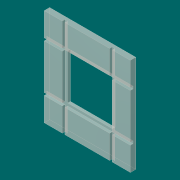
# Autodesk Inventor part: back
Saved by Autodesk Inventor 2016 (Build 200138000, 138)
## iProperties
Created: 2015-10-13
Part Number: back
Material: PC/ABS Plastic
Document SubType Name: Modeling
Designer: Sawaiz
Density: 0.357273 g/cm^3
Appearance: Clear
Author: Sawaiz
Autodesk Inventor part; units mm, degrees
ref_plane "YZ Plane" through (0, 0, 0) normal (1, 0, 0) x (0, 1, 0)
ref_plane "XZ Plane" through (0, 0, 0) normal (0, 1, 0) x (-1, 0, 0)
ref_plane "XY Plane" through (0, 0, 0) normal (0, 0, 1) x (1, 0, 0)
sketch "Sketch1" plane through (0, 0, 0) normal (1, 0, 0) x (0, 1, 0)
  line L0 (-50, -56.35) -> (50, -56.35)
  line L1 (50, -56.35) -> (50, 56.35)
  line L2 (50, 56.35) -> (-50, 56.35)
  line L3 (-50, 56.35) -> (-50, -56.35)
  line L4 (-50, -56.35) -> (50, 56.35) construction
  line L5 (50, -56.35) -> (-50, 56.35) construction
  point P0 (0, 0)
  dimension "d0" = 100
  dimension "d1" = 112.7
  constraints: 12 end point, 2 midpoint, 2 parallel, 1 horizontal, 1 perpendicular
  measures "d0" distance of L2.end L1.end
  measures "d1" distance of L1.end L0.end
extrude "Extrusion1" add sketch "Sketch1" along normal blind 6.35
sketch "Sketch2" plane through (6.35, 0, 0) normal (1, 0, 0) x (0, 0, -1)
  line L0 (-26, 26) -> (26, 26)
  line L1 (26, 26) -> (26, -26)
  line L2 (26, -26) -> (-26, -26)
  line L3 (-26, -26) -> (-26, 26)
  line L4 (-26, 26) -> (26, -26) construction
  line L5 (26, 26) -> (-26, -26) construction
  point P0 (0, 0)
  dimension "d4" = 52
  dimension "d5" = 52
  constraints: 12 end point, 2 midpoint, 2 parallel, 1 horizontal, 1 perpendicular
  measures "d4" distance of L1.end L2.end
  measures "d5" distance of L0.end L1.end
extrude "Extrusion2" cut sketch "Sketch2" against normal through all
sketch "Sketch3" plane through (6.35, 0, 0) normal (1, 0, 0) x (0, 0, -1)
  line L0 (-26, -26) -> (-26, 26) projected
  line L1 (-26, 26) -> (26, 26) projected
  line L2 (26, 26) -> (26, -26) projected
  line L3 (26, -26) -> (-26, -26) projected
  line L4 (56.35, -50) -> (56.35, 50) projected
  line L5 (56.35, 50) -> (-56.35, 50) projected
  line L6 (-56.35, 50) -> (-56.35, -50) projected
  line L7 (-56.35, -50) -> (56.35, -50) projected
  line L8 (-56.35, 29) -> (56.35, 29)
  line L9 (56.35, 29) -> (56.35, 26)
  line L10 (56.35, 26) -> (-56.35, 26)
  line L11 (-56.35, 26) -> (-56.35, 29)
  line L12 (-56.35, 29) -> (56.35, 26) construction
  line L13 (56.35, 29) -> (-56.35, 26) construction
  line L14 (-56.35, -29) -> (56.35, -29)
  line L15 (56.35, -29) -> (56.35, -26)
  line L16 (56.35, -26) -> (-56.35, -26)
  line L17 (-56.35, -26) -> (-56.35, -29)
  line L18 (-56.35, -29) -> (56.35, -26) construction
  line L19 (56.35, -29) -> (-56.35, -26) construction
  line L20 (56.35, 50) -> (-56.35, 50) projected
  line L21 (-29, 50) -> (-26, 50)
  line L22 (-26, 50) -> (-26, -50)
  line L23 (-26, -50) -> (-29, -50)
  line L24 (-29, -50) -> (-29, 50)
  line L25 (-56.35, -50) -> (56.35, -50) projected
  line L26 (26, -50) -> (29, -50)
  line L27 (29, -50) -> (29, 50)
  line L28 (29, 50) -> (26, 50)
  line L29 (26, 50) -> (26, -50)
  point P0 (0, 27.5)
  point P1 (0, -27.5)
  dimension "d12" = 3
  dimension "d13" = 3
  dimension "d14" = 3
  dimension "d15" = 3
  constraints: 40 end point, 8 parallel, 6 collinear, 6 point on line, 4 horizontal, 4 midpoint, 4 perpendicular
  measures "d12" distance between parallel lines of L14 L16
  measures "d13" distance between parallel lines of L8 L10
  measures "d14" distance between parallel lines of L22 L24
  measures "d15" distance between parallel lines of L27 L29
extrude "Extrusion3" cut sketch "Sketch3" against normal blind 3.175 contours L16 L24 L10 L0 | L22 L14 L24 L16 | L3 L29 L14 L22 | L22 L8 L29 L1 | L10 L24 L8 L22 | L2 L10 L27 L16 | L16 L27 L14 L29 | L24 L14 L6 L16 | L22 L7 L24 L14 | L29 L8 L27 L10 | L10 L6 L8 L24 | L8 L24 L5 L22 | L16 L4 L14 L27 | L14 L27 L7 L29 | L27 L8 L4 L10 | L29 L5 L27 L8
equation "\"d0\" = width"
equation "\"d1\" = height + 2 * acrylicThickness"
equation "\"d2\" = acrylicThickness"
equation "\"d4\" = detectorHeight"
equation "\"d5\" = detectorWidth"
equation "\"d12\" = mirrorThickness"
equation "\"d13\" = mirrorThickness"
equation "\"d14\" = mirrorThickness"
equation "\"d15\" = mirrorThickness"
equation "\"d10\" = 0.5 * acrylicThickness"
equation "\"acrylicThickness\" = 6.35"
equation "\"width\" = 100"
equation "\"mirrorAngle\" = 12deg"
equation "\"detectorWidth\" = 52"
equation "\"detectorHeight\" = 52"
equation "\"mirrorThickness\" = 3"
equation "\"fresnelThickness\" = 0.1"
equation "\"ior\" = 1.49"
equation "\"focalLength\" = 76.2"
equation "\"fresnelAngle\" = 90deg"
equation "\"centerThickness\" = 1.524"
equation "\"fresnelEffectiveDiameter\" = 76.2"
equation "\"height\" = 100"
body "Solid1"
